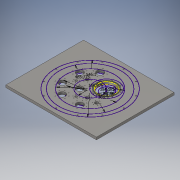
# Autodesk Inventor part: Top Plate V2
Saved by Autodesk Inventor 2018 (Build 220112000, 112)
## iProperties
Created: 2018-08-07
Part Number: Top Plate V2
Material: Stainless Steel, Austenitic
Document SubType Name: Modeling
Designer: freyja
Density: 8 g/cm^3
Appearance: Semi-Polished
Mass: 52241 g
Surface Area: 7917.75 cm^2
Volume: 6530.12 cm^3
Author: freyja
Autodesk Inventor part; units mm, degrees
ref_plane "YZ Plane" through (0, 0, 0) normal (1, 0, 0) x (0, 1, 0)
ref_plane "XZ Plane" through (0, 0, 0) normal (0, 1, 0) x (-1, 0, 0)
ref_plane "XY Plane" through (0, 0, 0) normal (0, 0, 1) x (1, 0, 0)
sketch "Sketch1" plane through (0, 0, 0) normal (0, 1, 0) x (-1, 0, 0)
  line L0 (355.6, 304.8) -> (-355.6, 304.8)
  line L1 (-355.6, 304.8) -> (-355.6, -304.8)
  line L2 (-355.6, -304.8) -> (355.6, -304.8)
  line L3 (355.6, -304.8) -> (355.6, 304.8)
  line L4 (355.6, 304.8) -> (-355.6, -304.8) construction
  line L5 (-355.6, 304.8) -> (355.6, -304.8) construction
  point P0 (0, 0)
  dimension "d0" = 711.2
  dimension "d1" = 609.6
  constraints: 12 end point, 2 midpoint, 2 parallel, 1 horizontal, 1 perpendicular
  measures "d0" distance of L2.end L1.end
  measures "d1" distance of L1.end L0.end
extrude "Extrusion1" add sketch "Sketch1" along normal blind 19.05
sketch "Sketch23" plane through (0, 19.05, 0) normal (0, 1, 0) x (1, 0, 0)
  circle A0 centre (0, 0) radius 273.05
  circle A1 centre (0, 0) radius 242.8875
  circle A2 centre (0, 0) radius 90.4875
  circle A3 centre (0, 0) radius 192.0875
  dimension "d167" = 546.1
  dimension "d168" = 485.775
  dimension "d292" = 180.975
  dimension "d293" = 384.175
  constraints: 4 centre point, 4 coincident
  measures "d167" diameter of A0
  measures "d168" diameter of A1
  measures "d292" diameter of A2
  measures "d293" diameter of A3
sketch "Sketch2" plane through (0, 19.05, 0) normal (0, 1, 0) x (1, 0, 0)
  line L0 (0, 0) -> (64.6578, 64.6578) construction
  line L1 (0, 0) -> (91.44, 0) construction
  circle A0 centre (64.6578, 64.6578) radius 118.745 construction
  circle A1 centre (64.6578, 64.6578) radius 68.58
  dimension "d4" = 91.44
  dimension "d5" = 45
  dimension "d6" = 237.49
  dimension "d7" = 137.16
  constraints: 4 end point, 2 centre point, 2 coincident, 1 equal length, 1 horizontal
  measures "d4" distance of L0.start L0.end
  measures "d5" angle of L1 L0
  measures "d6" diameter of A0
  measures "d7" diameter of A1
extrude "Extrusion2" cut sketch "Sketch2" against normal up to surface (19.05 mm away)
sketch "Sketch3" plane through (0, 19.05, 0) normal (0, 1, 0) x (1, 0, 0)
  circle A0 centre (64.6578, 64.6578) radius 68.58 projected
  line L0 (64.6578, 64.6578) -> (144.4441, 31.6093) construction
  line L1 (64.6578, 64.6578) -> (144.4441, 97.7064) construction
  line L2 (64.6578, 64.6578) -> (97.7064, 144.4441) construction
  line L3 (64.6578, 64.6578) -> (31.6093, 144.4441) construction
  line L4 (64.6578, 64.6578) -> (-15.1284, 97.7064) construction
  line L5 (64.6578, 64.6578) -> (-15.1284, 31.6093) construction
  line L6 (64.6578, 64.6578) -> (31.6093, -15.1284) construction
  line L7 (64.6578, 64.6578) -> (97.7064, -15.1284) construction
  line L8 (64.6578, 64.6578) -> (111.5909, 45.2175) construction
  line L9 (64.6578, 64.6578) -> (115.4578, 64.6578) construction
  point P0 (0, 0)
  dimension "d10" = 86.36
  dimension "d14" = 360
  dimension "d408" = 50.8
  dimension "d409" = 22.5
  constraints: 20 end point, 2 coincident, 1 collinear, 1 equal length, 1 horizontal, 23 other
  measures "d10" distance of L0.start L0.end
  measures "d408" distance of L7.start L8.end
  measures "d409" angle of L8 L9
hole "Hole1" at (144.4441, 19.05, -31.6093) at (144.4441, 19.05, -97.7064) at (97.7064, 19.05, -144.4441) at (31.6093, 19.05, -144.4441) at (-15.1284, 19.05, -97.7064) at (-15.1284, 19.05, -31.6093) at (31.6093, 19.05, 15.1284) at (97.7064, 19.05, 15.1284) direction (0, -1, 0) diameter 6.4008 depth 12.7 tip angle 118 thread size "5/16-18 UNC" class "2B" standard "ANSI Unified Screw Threads"
sketch "Sketch58" plane through (0, 19.05, 0) normal (0, 1, 0) x (1, 0, 0)
  circle A0 centre (64.6578, 64.6578) radius 68.58 projected
  circle A1 centre (64.6578, 64.6578) radius 93.98
  point P0 (0, 0)
  dimension "d495" = 187.96
  constraints: 1 centre point, 1 coincident
  measures "d495" diameter of A1
sketch "Sketch38" plane through (0, 19.05, 0) normal (0, 1, 0) x (1, 0, 0)
  circle A0 centre (64.6578, 64.6578) radius 68.58 projected
  circle A1 centre (64.6578, 64.6578) radius 75.9968
  circle A2 centre (64.6578, 64.6578) radius 80.01
  point P0 (0, 0)
  dimension "d288" = 151.9936
  dimension "d289" = 160.02
  constraints: 2 centre point, 2 coincident
  measures "d288" diameter of A1
  measures "d289" diameter of A2
extrude "Extrusion22" cut sketch "Sketch38" against normal blind 3.175 contours A2
sketch "Sketch4" plane through (0, 19.05, 0) normal (0, 1, 0) x (1, 0, 0)
  line L0 (0, 0) -> (-149.6314, -69.7743) construction
  line L1 (0, 0) -> (165.1, 0) construction
  circle A0 centre (-149.6314, -69.7743) radius 26.289
  dimension "d23" = 165.1
  dimension "d24" = 205
  dimension "d25" = 52.578
  constraints: 4 end point, 1 centre point, 1 coincident, 1 equal length, 1 horizontal
  measures "d23" distance of L0.start L0.end
  measures "d25" diameter of A0
extrude "Extrusion3" cut sketch "Sketch4" against normal up to surface (19.05 mm away)
sketch "Sketch6" plane through (0, 19.05, 0) normal (0, 1, 0) x (1, 0, 0)
  circle A0 centre (-149.6314, -69.7743) radius 24.13 construction
  line L0 (-149.6314, -69.7743) -> (-111.4983, -85.5695) construction
  line L1 (-149.6314, -69.7743) -> (-108.3564, -69.7743) construction
  line L2 (-149.6314, -69.7743) -> (-111.4983, -53.979) construction
  line L3 (-149.6314, -69.7743) -> (-133.8362, -31.6411) construction
  line L4 (-149.6314, -69.7743) -> (-165.4267, -31.6411) construction
  line L5 (-149.6314, -69.7743) -> (-187.7645, -53.979) construction
  line L6 (-149.6314, -69.7743) -> (-187.7645, -85.5695) construction
  line L7 (-149.6314, -69.7743) -> (-165.4267, -107.9074) construction
  line L8 (-149.6314, -69.7743) -> (-133.8362, -107.9074) construction
  line L9 (-149.6314, -69.7743) -> (-137.8981, -74.6344) construction
  line L10 (-149.6314, -69.7743) -> (-136.9314, -69.7743) construction
  point P0 (0, 0)
  dimension "d31" = 41.275
  dimension "d35" = 360
  dimension "d404" = 12.7
  dimension "d405" = 22.5
  constraints: 22 end point, 2 coincident, 2 horizontal, 1 collinear, 1 equal length, 23 other
  measures "d31" distance of L0.start L0.end
  measures "d404" distance of L8.start L9.end
  measures "d405" angle of L9 L10
hole "Hole2" at (-111.4983, 19.05, 53.979) at (-133.8362, 19.05, 31.6411) at (-165.4267, 19.05, 31.6411) at (-187.7645, 19.05, 53.979) at (-187.7645, 19.05, 85.5695) at (-165.4267, 19.05, 107.9074) at (-133.8362, 19.05, 107.9074) at (-111.4983, 19.05, 85.5695) direction (0, -1, 0) diameter 3.9624 depth 13.6144 tip angle 118 thread size "10-32 UNF" class "2B" standard "ANSI Unified Screw Threads"
pattern_circular "Circular Pattern1" count 3 over 180 about axis through (0, -10, 0) along (0, 1, 0) of "Extrusion3", "Hole2" both ways yes
sketch "Sketch7" plane through (0, 19.05, 0) normal (0, 1, 0) x (1, 0, 0)
  line L0 (0, 0) -> (50.9909, -72.8226) construction
  line L1 (0, 0) -> (88.9, 0) construction
  circle A0 centre (50.9909, -72.8226) radius 13.208
  dimension "d44" = 88.9
  dimension "d45" = 305
  dimension "d46" = 26.416
  constraints: 4 end point, 1 centre point, 1 coincident, 1 equal length, 1 horizontal
  measures "d44" distance of L0.start L0.end
  measures "d46" diameter of A0
extrude "Extrusion5" cut sketch "Sketch7" against normal up to surface (19.05 mm away)
sketch "Sketch51" plane through (0, 19.05, 0) normal (0, 1, 0) x (1, 0, 0)
  circle A0 centre (50.9909, -72.8226) radius 13.208 projected
  line L0 (50.9909, -72.8226) -> (74.9909, -72.8226)
  line L1 (50.9909, -72.8226) -> (74.9909, -72.8226) construction
  line L2 (50.9909, -72.8226) -> (62.9909, -52.038)
  line L3 (50.9909, -72.8226) -> (38.9909, -52.038)
  line L4 (50.9909, -72.8226) -> (26.9909, -72.8226)
  line L5 (50.9909, -72.8226) -> (38.9909, -93.6072)
  line L6 (50.9909, -72.8226) -> (62.9909, -93.6072)
  point P0 (0, 0)
  dimension "d423" = 24
  dimension "d424" = 0
  dimension "d427" = 360
  constraints: 14 end point, 2 coincident, 1 collinear, 1 horizontal, 17 other
  measures "d423" distance of L0.start L0.end
  measures "d424" distance between parallel lines of L1 L0
hole "Hole20" at (62.9909, 19.05, 52.038) at (38.9909, 19.05, 52.038) at (26.9909, 19.05, 72.8226) at (38.9909, 19.05, 93.6072) at (62.9909, 19.05, 93.6072) at (74.9909, 19.05, 72.8226) direction (0, -1, 0) diameter 3.9624 depth 13.6144 tip angle 118 thread size "10-32 UNF" class "2B" standard "ANSI Unified Screw Threads"
sketch "Sketch26" plane through (0, 19.05, 0) normal (0, 1, 0) x (1, 0, 0)
  line L0 (0, 0) -> (-107.95, 0) construction
  line L1 (0, 0) -> (107.95, 0) construction
  circle A0 centre (-107.95, 0) radius 8.636
  dimension "d185" = 107.95
  dimension "d186" = 180
  dimension "d187" = 17.272
  constraints: 4 end point, 1 centre point, 1 coincident, 1 collinear, 1 horizontal
  measures "d185" distance of L0.start L0.end
  measures "d186" angle of L0 L1
  measures "d187" diameter of A0
extrude "Extrusion16" cut sketch "Sketch26" against normal up to surface (19.05 mm away)
sketch "Sketch28" plane through (0, 19.05, 0) normal (0, 1, 0) x (1, 0, 0)
  circle A0 centre (-107.95, 0) radius 8.636 projected
  line L0 (-107.95, 0) -> (-127, 0) construction
  line L1 (-107.95, 0) -> (-88.9, 0) construction
  line L2 (-107.95, 0) -> (-117.475, -16.4978) construction
  line L3 (-107.95, 0) -> (-98.425, -16.4978) construction
  line L4 (-107.95, 0) -> (-88.9, 0) construction
  line L5 (-107.95, 0) -> (-98.425, 16.4978) construction
  line L6 (-107.95, 0) -> (-117.475, 16.4978) construction
  point P0 (0, 0)
  dimension "d193" = 19.05
  dimension "d194" = 180
  dimension "d204" = 360
  constraints: 14 end point, 2 coincident, 2 horizontal, 1 collinear, 17 other
  measures "d193" distance of L0.start L0.end
  measures "d194" angle of L0 L1
hole "Hole9" at (-127, 19.05, 0) at (-117.475, 19.05, -16.4978) at (-98.425, 19.05, -16.4978) at (-88.9, 19.05, 0) at (-98.425, 19.05, 16.4978) at (-117.475, 19.05, 16.4978) direction (0, -1, 0) diameter 3.9624 depth 13.6144 tip angle 118 thread size "10-32 UNF" class "2B" standard "ANSI Unified Screw Threads"
pattern_circular "Circular Pattern6" count 2 over 90 about axis through (0, -10, 0) along (0, 1, 0) of "Extrusion16", "Hole9"
sketch "Sketch30" plane through (0, 19.05, 0) normal (0, 1, 0) x (1, 0, 0)
  line L0 (0, 0) -> (-69.7743, -149.6314) construction
  line L1 (0, 0) -> (165.1, 0) construction
  circle A0 centre (-69.7743, -149.6314) radius 26.289
  dimension "d221" = 165.1
  dimension "d222" = 115
  dimension "d223" = 52.578
  constraints: 4 end point, 1 centre point, 1 coincident, 1 equal length, 1 horizontal
  measures "d221" distance of L0.start L0.end
  measures "d222" angle of L0 L1
  measures "d223" diameter of A0
extrude "Extrusion18" cut sketch "Sketch30" against normal up to surface (19.05 mm away)
sketch "Sketch32" plane through (0, 19.05, 0) normal (0, 1, 0) x (1, 0, 0)
  circle A0 centre (-69.7743, -149.6314) radius 26.289 construction
  line L0 (-69.7743, -149.6314) -> (-107.9074, -133.8362) construction
  line L1 (-69.7743, -149.6314) -> (-107.9074, -165.4267) construction
  line L2 (-69.7743, -149.6314) -> (-85.5695, -187.7645) construction
  line L3 (-69.7743, -149.6314) -> (-53.979, -187.7645) construction
  line L4 (-69.7743, -149.6314) -> (-31.6411, -165.4267) construction
  line L5 (-69.7743, -149.6314) -> (-31.6411, -133.8362) construction
  line L6 (-69.7743, -149.6314) -> (-53.979, -111.4983) construction
  line L7 (-69.7743, -149.6314) -> (-85.5695, -111.4983) construction
  line L8 (-69.7743, -149.6314) -> (-58.041, -154.4915) construction
  line L9 (-69.7743, -149.6314) -> (-57.0743, -149.6314) construction
  point P0 (0, 0)
  dimension "d229" = 41.275
  dimension "d232" = 360
  dimension "d406" = 12.7
  dimension "d407" = 22.5
  constraints: 20 end point, 2 coincident, 1 collinear, 1 equal length, 1 horizontal, 23 other
  measures "d229" distance of L0.start L0.end
  measures "d406" distance of L7.start L8.end
  measures "d407" angle of L8 L9
hole "Hole10" at (-85.5695, 19.05, 111.4983) at (-107.9074, 19.05, 133.8362) at (-53.979, 19.05, 111.4983) at (-31.6411, 19.05, 133.8362) at (-31.6411, 19.05, 165.4267) at (-53.979, 19.05, 187.7645) at (-85.5695, 19.05, 187.7645) at (-107.9074, 19.05, 165.4267) direction (0, -1, 0) diameter 3.9624 depth 13.6144 tip angle 118 thread size "10-32 UNF" class "2B" standard "ANSI Unified Screw Threads"
pattern_circular "Circular Pattern7" count 2 over 90 about axis through (0, -10, 0) along (0, -1, 0) of "Extrusion18", "Hole10" both ways yes
sketch "Sketch37" plane through (0, 19.05, 0) normal (0, 1, 0) x (1, 0, 0)
  line L0 (0, 0) -> (-265.25, 0)
  dimension "d277" = 265.25
  constraints: 2 end point, 1 horizontal
  measures "d277" distance of L0.start L0.end
hole "Hole13" at (-265.25, 19.05, 0) direction (0, -1, 0) diameter 8.9916 depth 21.1074 tip angle 118 clearance for "Socket Head Cap Screw" size "M8" standard "Ansi Metric M Profile"
pattern_circular "Circular Pattern9" count 12 over 360 about axis through (0, -10, 0) along (0, 1, 0) of "Hole13"
sketch "Sketch39" plane through (0, 19.05, 0) normal (0, 1, 0) x (1, 0, 0)
  line L0 (0, 0) -> (-40.4112, -40.4112) construction
  line L1 (0, 0) -> (57.15, 0) construction
  circle A0 centre (-40.4112, -40.4112) radius 26.289
  dimension "d294" = 57.15
  dimension "d295" = 135
  dimension "d296" = 52.578
  constraints: 4 end point, 1 centre point, 1 coincident, 1 equal length, 1 horizontal
  measures "d294" distance of L0.start L0.end
  measures "d295" angle of L0 L1
  measures "d296" diameter of A0
extrude "Extrusion23" cut sketch "Sketch39" against normal up to surface (19.05 mm away)
sketch "Sketch50" plane through (0, 19.05, 0) normal (0, 1, 0) x (1, 0, 0)
  circle A0 centre (-40.4112, -40.4112) radius 26.289 construction
  line L0 (-40.4112, -40.4112) -> (0.8638, -40.4112) construction
  line L1 (-40.4112, -40.4112) -> (0.8638, -40.4112) construction
  line L2 (-40.4112, -40.4112) -> (-11.2253, -11.2253) construction
  line L3 (-40.4112, -40.4112) -> (-40.4112, 0.8638) construction
  line L4 (-40.4112, -40.4112) -> (-69.597, -11.2253) construction
  line L5 (-40.4112, -40.4112) -> (-81.6862, -40.4112) construction
  line L6 (-40.4112, -40.4112) -> (-69.597, -69.597) construction
  line L7 (-40.4112, -40.4112) -> (-40.4112, -81.6862) construction
  line L8 (-40.4112, -40.4112) -> (-11.2253, -69.597) construction
  point P0 (0, 0)
  dimension "d410" = 41.275
  dimension "d411" = 0
  dimension "d414" = 360
  constraints: 18 end point, 2 coincident, 1 collinear, 1 horizontal, 23 other
  measures "d410" distance of L0.start L0.end
  measures "d411" distance between parallel lines of L1 L0
hole "Hole19" at (0.8638, 19.05, 40.4112) at (-11.2253, 19.05, 11.2253) at (-40.4112, 19.05, -0.8638) at (-69.597, 19.05, 11.2253) at (-69.597, 19.05, 69.597) at (-40.4112, 19.05, 81.6862) at (-11.2253, 19.05, 69.597) at (-81.6862, 19.05, 40.4112) direction (0, -1, 0) diameter 3.9624 depth 13.6144 tip angle 118 thread size "10-32 UNF" class "2B" standard "ANSI Unified Screw Threads"
pattern_circular "Circular Pattern11" count 2 over 200 about axis through (0, -10, 0) along (0, 1, 0) of "Extrusion5"
sketch "Sketch45" plane through (0, 19.05, 0) normal (0, 1, 0) x (1, 0, 0)
  line L0 (0, 0) -> (123.1835, -71.12) construction
  line L1 (0, 0) -> (142.24, 0) construction
  circle A0 centre (123.1835, -71.12) radius 13.208
  dimension "d349" = 142.24
  dimension "d350" = 30
  dimension "d351" = 26.416
  constraints: 4 end point, 1 centre point, 1 coincident, 1 equal length, 1 horizontal
  measures "d349" distance of L0.start L0.end
  measures "d350" angle of L0 L1
  measures "d351" diameter of A0
extrude "Extrusion27" cut sketch "Sketch45" against normal up to surface (19.05 mm away)
sketch "Sketch54" plane through (0, 19.05, 0) normal (0, 1, 0) x (1, 0, 0)
  circle A0 centre (123.1835, -71.12) radius 13.208 projected
  line L0 (123.1835, -71.12) -> (143.9681, -59.12)
  line L1 (123.1835, -71.12) -> (147.1835, -71.12) construction
  line L2 (123.1835, -71.12) -> (123.1835, -47.12)
  line L3 (123.1835, -71.12) -> (102.3988, -59.12)
  line L4 (123.1835, -71.12) -> (102.3988, -83.12)
  line L5 (123.1835, -71.12) -> (123.1835, -95.12)
  line L6 (123.1835, -71.12) -> (143.9681, -83.12)
  point P0 (0, 0)
  dimension "d461" = 24
  dimension "d462" = 30
  dimension "d465" = 360
  constraints: 14 end point, 2 coincident, 1 equal length, 1 horizontal, 17 other
  measures "d461" distance of L0.start L0.end
  measures "d462" angle of L1 L0
hole "Hole23" at (143.9681, 19.05, 59.12) at (123.1835, 19.05, 47.12) at (102.3988, 19.05, 59.12) at (102.3988, 19.05, 83.12) at (143.9681, 19.05, 83.12) at (123.1835, 19.05, 95.12) direction (0, -1, 0) diameter 3.9624 depth 13.6144 tip angle 118 thread size "10-32 UNF" class "2B" standard "ANSI Unified Screw Threads"
sketch "Sketch49" plane through (0, 0, 0) normal (0, -1, 0) x (1, 0, 0)
  line L0 (0, 0) -> (165.1, 0) construction
  line L1 (0, 0) -> (165.1, 0) construction
  line L2 (165.1, 0) -> (152.4, 0) construction
  line L3 (165.1, 0) -> (183.0605, 17.9605) construction
  line L4 (165.1, 0) -> (190.5, 0) construction
  line L5 (165.1, 0) -> (147.1395, 17.9605) construction
  line L6 (165.1, 0) -> (147.1395, -17.9605) construction
  line L7 (165.1, 0) -> (183.0605, -17.9605) construction
  dimension "d384" = 165.1
  dimension "d385" = 0
  dimension "d388" = 25.4
  dimension "d389" = 45
  dimension "d392" = 360
  constraints: 16 end point, 3 horizontal, 2 equal length, 13 other
  measures "d384" distance of L0.start L0.end
  measures "d385" distance between parallel lines of L1 L0
  measures "d388" distance of L1.end L3.end
  measures "d389" angle of L4 L3
hole "Hole18" at (183.0605, 0, -17.9605) at (147.1395, 0, -17.9605) at (147.1395, 0, 17.9605) at (183.0605, 0, 17.9605) direction (0, 1, 0) diameter 4.3434 depth 16.256 tip angle 118 thread size "12-24 UNC" class "2B" standard "ANSI Unified Screw Threads"
pattern_circular "Circular Pattern12" count 4 over 360 about axis through (0, -10, 0) along (0, 1, 0) of "Hole18"
sketch "Sketch53" plane through (0, 19.05, 0) normal (0, 1, 0) x (1, 0, 0)
  circle A0 centre (-72.8226, 50.9909) radius 13.208 projected
  line L0 (-72.8226, 50.9909) -> (-50.5702, 59.9815)
  line L1 (-72.8226, 50.9909) -> (-48.8226, 50.9909) construction
  line L2 (-72.8226, 50.9909) -> (-69.4825, 74.7574)
  line L3 (-72.8226, 50.9909) -> (-91.7349, 65.7668)
  line L4 (-72.8226, 50.9909) -> (-95.075, 42.0004)
  line L5 (-72.8226, 50.9909) -> (-76.1628, 27.2245)
  line L6 (-72.8226, 50.9909) -> (-53.9104, 36.2151)
  point P0 (0, 0)
  dimension "d448" = 24
  dimension "d449" = 22
  dimension "d452" = 360
  constraints: 14 end point, 2 coincident, 1 equal length, 1 horizontal, 17 other
  measures "d448" distance of L0.start L0.end
  measures "d449" angle of L1 L0
hole "Hole22" at (-50.5702, 19.05, -59.9815) at (-69.4825, 19.05, -74.7574) at (-91.7349, 19.05, -65.7668) at (-95.075, 19.05, -42.0004) at (-76.1628, 19.05, -27.2245) at (-53.9104, 19.05, -36.2151) direction (0, -1, 0) diameter 3.9624 depth 13.6144 tip angle 118 thread size "10-32 UNF" class "2B" standard "ANSI Unified Screw Threads"
sketch "Sketch55" plane through (0, 0, 0) normal (0, -1, 0) x (1, 0, 0)
  circle A0 centre (-40.4112, 40.4112) radius 26.289 projected
  line L0 (-40.4112, 40.4112) -> (-2.278, 56.2064)
  line L1 (-40.4112, 40.4112) -> (0.8638, 40.4112) construction
  line L2 (-40.4112, 40.4112) -> (-24.6159, 78.5443)
  line L3 (-40.4112, 40.4112) -> (-56.2064, 78.5443)
  line L4 (-40.4112, 40.4112) -> (-78.5443, 56.2064)
  line L5 (-40.4112, 40.4112) -> (-78.5443, 24.6159)
  line L6 (-40.4112, 40.4112) -> (-56.2064, 2.278)
  line L7 (-40.4112, 40.4112) -> (-24.6159, 2.278)
  line L8 (-40.4112, 40.4112) -> (-2.278, 24.6159)
  point P0 (0, 0)
  dimension "d474" = 41.275
  dimension "d475" = 22.5
  dimension "d478" = 360
  constraints: 18 end point, 2 coincident, 1 equal length, 1 horizontal, 23 other
  measures "d474" distance of L0.start L0.end
  measures "d475" angle of L1 L0
hole "Hole24" at (-24.6159, 0, 78.5443) at (-2.278, 0, 56.2064) at (-56.2064, 0, 78.5443) at (-78.5443, 0, 56.2064) at (-78.5443, 0, 24.6159) at (-56.2064, 0, 2.278) at (-24.6159, 0, 2.278) at (-2.278, 0, 24.6159) direction (0, 1, 0) diameter 3.9624 depth 13.6144 tip angle 118 thread size "10-32 UNF" class "2B" standard "ANSI Unified Screw Threads"
sketch "Sketch56" plane through (0, 19.05, 0) normal (0, 1, 0) x (1, 0, 0)
  circle A0 centre (64.6578, 64.6578) radius 68.58 projected
  circle A1 centre (64.6578, 64.6578) radius 69.85
  circle A2 centre (64.6578, 64.6578) radius 73.025
  point P0 (0, 0)
  dimension "d487" = 139.7
  dimension "d488" = 146.05
  constraints: 2 centre point, 2 coincident
  measures "d487" diameter of A1
  measures "d488" diameter of A2
extrude "Extrusion29" cut sketch "Sketch56" against normal blind 1.5875 contours A2
sketch "Sketch57" plane through (0, 0, 0) normal (0, -1, 0) x (1, 0, 0)
  circle A0 centre (0, 0) radius 142.875
  circle A1 centre (0, 0) radius 184.15
  circle A2 centre (64.6578, -64.6578) radius 68.58 projected
  circle A3 centre (64.6578, -64.6578) radius 64.77
  circle A4 centre (64.6578, -64.6578) radius 46.99
  dimension "d491" = 285.75
  dimension "d492" = 368.3
  dimension "d493" = 129.54
  dimension "d494" = 93.98
  constraints: 4 centre point, 4 coincident
  measures "d491" diameter of A0
  measures "d492" diameter of A1
  measures "d493" diameter of A3
  measures "d494" diameter of A4
body "Solid1"
